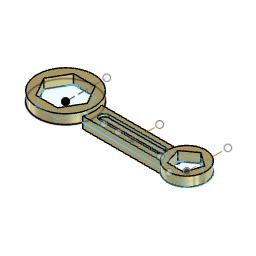
Ex2 (Autodesk Fusion 360 design; units mm, degrees)
Autodesk Fusion 360 part; units mm, degrees
sketch "Sketch1" plane through (0, 0, 0) normal (0, 0, 1) x (1, 0, 0) in component "ex2"
  circle A0 centre (0, 0) radius 30
  circle A1 centre (129, 0) radius 20
  line L0 (0, 0) -> (0, 43.8518) construction
  line L1 (129, 0) -> (129, 43.6821) construction
  line L2 (-11.547, 20) -> (-23.094, 0)
  line L3 (-23.094, 0) -> (-11.547, -20)
  line L4 (-11.547, -20) -> (11.547, -20)
  line L5 (11.547, -20) -> (23.094, 0)
  line L6 (23.094, 0) -> (11.547, 20)
  line L7 (11.547, 20) -> (-11.547, 20)
  line L8 (129, 15) -> (114.7342, 4.6353)
  line L9 (114.7342, 4.6353) -> (120.1832, -12.1353)
  line L10 (120.1832, -12.1353) -> (137.8168, -12.1353)
  line L11 (137.8168, -12.1353) -> (143.2658, 4.6353)
  line L12 (143.2658, 4.6353) -> (129, 15)
  line L13 (28.2843, 10) -> (111.6795, 10)
  line L14 (49.2985, 10) -> (49.2985, -10) construction
  line L15 (49.2985, 0) -> (56, 0) construction
  line L16 (28.2843, -10) -> (111.6795, -10)
  line L17 (119.4894, -10) -> (120.196, -10)
  line L18 (30, 0) -> (109, 0)
  line L19 (71.1993, 0) -> (71.1993, 28.9403) construction
  line L20 (101.1993, 5) -> (41.1993, 5)
  line L21 (41.1993, -5) -> (101.1993, -5)
  line L22 (101.1993, 5) -> (41.1993, -5) construction
  line L23 (41.1993, 5) -> (101.1993, -5) construction
  arc A2 (42.8209, 4.7297) -> (42.8209, -4.7297) centre (41.1993, 0) ccw
  arc A3 (99.5777, -4.7297) -> (99.5777, 4.7297) centre (101.1993, 0) ccw
  point P0 (129, 0)
  point P1 (71.1993, 0)
  dimension "d9" = 60
  dimension "d10" = 40
  dimension "d11" = 129
  dimension "d12" = 20
  dimension "d13" = 15
  dimension "d14" = 10
  dimension "d15" = 10
  dimension "d16" = 60
  dimension "d17" = 10
  constraint coincident A0.centre L0.start
  constraint horizontal L18
  constraint coincident P0 A1.centre
  constraint vertical L1
  constraint vertical L0
  constraint coincident L1 L8.start
  constraint horizontal L13
  constraint horizontal L16
  constraint coincident L13 L14.start
  constraint coincident L14.end L16
  constraint vertical L14
  constraint coincident L14 L15.start
  constraint perpendicular L14 L15
  constraint collinear L15 L18
  constraint coincident A0 L13.start
  constraint coincident A0 L18.start
  constraint coincident A0 L16.start
  constraint coincident A1 L16.end
  constraint coincident L9 L17.start
  constraint collinear L16 L17
  constraint coincident A1 L18.end
  constraint coincident A1 L13.end
  constraint coincident L18 P1
  constraint vertical L19
  constraint horizontal L20
  constraint parallel L20 L21
  constraint coincident L22 P1
  constraint coincident L23 P1
  constraint coincident P1 L19.start
  constraint coincident L20.end A2
  constraint tangent L20 A2
  constraint coincident L21.start A2
  constraint coincident L20.start A3
  constraint tangent L20 A3
  constraint coincident L21.end A3
  constraint coincident L23 A2.start
  constraint coincident L22 A2.end
  constraint coincident L23 A3.start
  constraint coincident L22 A3.end
  measures "d9" diameter of A0
  measures "d10" diameter of A1
  measures "d11" distance of A0.centre P0
  measures "d12" distance of A0.centre L7
  measures "d13" distance of L8.start P0
  measures "d14" distance of L13 L18
  measures "d15" distance of L16 L18
  measures "d16" distance of L21.start L21.end
  measures "d17" distance of L20.end L21.start
extrude "Extrude1" add sketch "Sketch1" along normal blind 10 contours A0 | A1 makes body 1 at (29.8509, 2.987, 6.6667) makes body 2 at (148.9006, -1.9914, 3.3333) in component "ex2"
extrude "Extrude2" add sketch "Sketch1" along normal mid plane 12 contours A0 A1 L16 L18 L21 A2 A3 | A0 A1 L13 L18 L20 A2 A3 bodies 1 2 in component "ex2"
extrude "Extrude3" add sketch "Sketch1" along normal mid plane 6 contours L18 L20 A2 A3 bodies 1 in component "ex2"
component "ex2" placed x (1, 0, 0) y (0, 1, 0) z (0, 0, 1) at (0, 0, 0)
